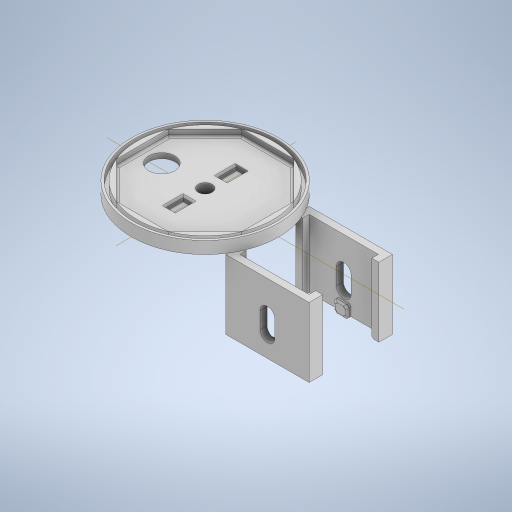
# Autodesk Inventor part: Bi_PAM
Saved by Autodesk Inventor 2024 (Build 280153000, 153)
## iProperties
Created: 2023-07-24
Part Number: Bi_PAM
Material: 일반
Document SubType Name: Modeling
Designer: jsw
Density: 1 g/cm^3
Appearance: 기본값
Author: jsw
Autodesk Inventor part; units mm, degrees
ref_plane "YZ Plane" through (0, 0, 0) normal (1, 0, 0) x (0, 1, 0)
sketch "스케치1" plane through (0, 0, 0) normal (0, 1, 0) x (-1, 0, 0)
  circle A0 centre (0, 0) radius 39
  circle A1 centre (0, 0) radius 42.5
  dimension "d0" = 78
  dimension "d6" = 3.5
  constraints: 2 centre point, 2 coincident
  measures "d0" diameter of A0
  measures "d6" radial gap between concentric circles of A0 A1
extrude "돌출1" add sketch "스케치1" along normal blind 7 contours A0 | A1
sketch "스케치4" plane through (0, 7, 0) normal (0, 1, 0) x (1, 0, 0)
  line L0 (15, -36.2132) -> (-15, -36.2132)
  line L1 (-15, -36.2132) -> (-36.2132, -15)
  line L2 (-36.2132, -15) -> (-36.2132, 15)
  line L3 (-36.2132, 15) -> (-15, 36.2132)
  line L4 (-15, 36.2132) -> (15, 36.2132)
  line L5 (15, 36.2132) -> (36.2132, 15)
  line L6 (36.2132, 15) -> (36.2132, -15)
  line L7 (36.2132, -15) -> (15, -36.2132)
  point P0 (0, 0)
  point P1 (0, 0)
  dimension "d17" = 30
  constraints: 16 end point, 1 coincident, 1 horizontal, 17 other
  measures "d17" distance of L0.start L0.end
extrude "돌출4" cut sketch "스케치4" against normal blind 4
fillet "모깎기1" radius 1.2 8 edges at (0, 3, -36.2132) (25.6066, 3, -25.6066) (36.2132, 3, 0) (25.6066, 3, 25.6066) (0, 3, 36.2132) (-25.6066, 3, 25.6066) (-36.2132, 3, 0) (-25.6066, 3, -25.6066)
sketch "스케치6" plane through (0, 7, 0) normal (0, 1, 0) x (1, 0, 0)
  line L0 (36.2132, -15) -> (36.2132, 15) projected
  circle A0 centre (0, 0) radius 39.1969
  circle A1 centre (0, 0) radius 41.1969
  dimension "d30" = 2
  constraints: 2 coincident, 1 centre point, 3 other
extrude "돌출6" cut sketch "스케치6" against normal blind 4
sketch "스케치9" plane through (0, 0, 0) normal (0, -1, 0) x (1, 0, 0)
  line L0 (80, -20) -> (40, -20)
  line L1 (40, -20) -> (40, 20)
  line L2 (40, 20) -> (80, 20)
  line L3 (80, 20) -> (80, -20)
  line L4 (80, -20) -> (40, 20) construction
  line L5 (40, -20) -> (80, 20) construction
  line L6 (84, -24) -> (36, -24)
  line L7 (36, -24) -> (36, 24)
  line L8 (36, 24) -> (84, 24)
  line L9 (84, 24) -> (84, -24)
  line L10 (84, -24) -> (36, 24) construction
  line L11 (36, -24) -> (84, 24) construction
  line L12 (0, -59.5) -> (0, 59.5) projected
  line L13 (-67.8, 0) -> (109.3, 0) projected
  point P0 (60, 0)
  point P1 (60, 0)
  dimension "d54" = 40
  dimension "d55" = 40
  dimension "d56" = 4
  dimension "d112" = 60
  dimension "d113" = 0
  constraints: 24 end point, 5 midpoint, 4 parallel, 2 horizontal, 2 perpendicular, 1 point on line
  measures "d54" distance of L1.end L2.end
  measures "d55" distance of L0.end L1.end
  measures "d56" distance between parallel lines of L2 L8
  measures "d112" distance from line of point (60, 0) L12
  measures "d113" distance from line of L13 point (60, 0)
extrude "돌출9" add sketch "스케치9" along normal blind 40 contours L3 L13 L9 L6 L7 L1 L0 | L3 L2 L1 L13 L7 L8 L9
ref_plane "작업 평면2" through (60, 0, 24) normal (1, 0, 0) x (0, 0, -1)
sketch "스케치11" plane through (36, 0, 24) normal (0, 0, 1) x (1, 0, 0)
  line L0 (24, -18.25) -> (24, -27.75) construction
  line L1 (19.75, -18.25) -> (19.75, -27.75)
  line L2 (28.25, -27.75) -> (28.25, -18.25)
  arc A0 (28.25, -18.25) -> (19.75, -18.25) centre (24, -18.25) ccw
  arc A1 (19.75, -27.75) -> (28.25, -27.75) centre (24, -27.75) ccw
  line L3 (0, 0) -> (48, 0) projected
  line L4 (48, 0) -> (0, 0) projected
  point P0 (-36, 0)
  point P1 (24, -23)
  point P2 (28.25, -23)
  point P3 (24, 0)
  point P4 (24, -32)
  point P5 (24, -14)
  dimension "d63" = 4.25
  dimension "d64" = 18
  dimension "d65" = 23
  constraints: 8 end point, 6 point on circle, 4 tangent, 3 midpoint, 2 centre point, 1 parallel, 1 vertical, 1 vertical alignment
  measures "d63" distance of point (28.25, -23) point (24, -23)
  measures "d64" distance of point (24, -32) point (24, -14)
  measures "d65" distance from line of L3 point (24, -23)
extrude "돌출11" cut sketch "스케치11" against normal up to surface (48 mm away)
sketch "스케치12" plane through (80, 0, 20) normal (0, 0, -1) x (-1, 0, 0)
  line L0 (40, -40) -> (0, -40) projected
  line L1 (16, -40) -> (24, -40)
  line L2 (24, -40) -> (24, -33)
  line L3 (24, -33) -> (16, -33)
  line L4 (16, -33) -> (16, -40)
  line L5 (15.75, -18.25) -> (15.75, -27.75) projected
  line L6 (15.75, -23) -> (24.25, -23)
  line L7 (24.25, -27.75) -> (24.25, -18.25) projected
  line L8 (40, -6) -> (0, -6)
  line L9 (24, -6) -> (24, -13)
  line L10 (24, -13) -> (16, -13)
  line L11 (16, -13) -> (16, -6)
  point P0 (80, 0)
  point P1 (20, -40)
  point P2 (20, -40)
  point P3 (24, -6)
  dimension "d68" = 8
  dimension "d69" = 7
  dimension "d70" = 0
  constraints: 18 end point, 6 symmetric about line, 4 midpoint, 2 parallel, 2 point on line, 1 horizontal, 1 perpendicular
  measures "d68" distance of L3.end L2.end
  measures "d69" distance of L1.end L2.end
  measures "d70" distance of point (20, -40) point (20, -40)
extrude "돌출12" add sketch "스케치12" along normal blind 2 contours L0 L4 L3 L2
fillet "모깎기3" radius 1 4 edges at (56, -36.5, 18) (64, -36.5, 18) (60, -33, 18) (60, -40, 18)
ref_plane "작업 평면3" through (84, 0, 0) normal (0, 0, -1) x (-1, 0, 0)
mirror "미러2" about plane through (84, 0, 0) normal (0, 0, -1) of "모깎기3", "돌출12"
sketch "스케치13" plane through (0, 3, 0) normal (0, 1, 0) x (1, 0, 0)
  line L0 (2.75, -21) -> (-2.75, -21)
  line L1 (-2.75, -21) -> (-2.75, -10)
  line L2 (-2.75, -10) -> (2.75, -10)
  line L3 (2.75, -10) -> (2.75, -21)
  line L4 (2.75, -21) -> (-2.75, -10) construction
  line L5 (-2.75, -21) -> (2.75, -10) construction
  line L6 (-35.9913, 0) -> (36.8765, 0)
  line L7 (2.75, 21) -> (-2.75, 21)
  line L8 (-2.75, 21) -> (-2.75, 10)
  line L9 (-2.75, 10) -> (2.75, 10)
  line L10 (2.75, 10) -> (2.75, 21)
  line L11 (2.75, 21) -> (-2.75, 10) construction
  line L12 (-2.75, 21) -> (2.75, 10) construction
  point P0 (0, 0)
  point P1 (0, -15.5)
  point P2 (0, -10)
  point P3 (0, 15.5)
  point P4 (0, 10)
  point P5 (0.4426, 0)
  dimension "d75" = 5.5
  dimension "d76" = 11
  dimension "d77" = 10
  dimension "d78" = 0
  constraints: 26 end point, 6 symmetric about line, 4 midpoint, 2 horizontal, 2 parallel, 1 perpendicular, 1 vertical alignment
  measures "d75" distance of L1.end L2.end
  measures "d76" distance of L0.end L1.end
  measures "d77" distance of point (0, -10) point (0, 0)
  measures "d78" vertical distance of point (0, 0) point (0.443, 0)
extrude "돌출13" cut sketch "스케치13" against normal up to surface (3 mm away)
sketch "스케치14" plane through (36, 0, -24) normal (-1, 0, 0) x (0, 0, 1)
  line L0 (66.5, 0) -> (-18.5, 0) projected
  circle A0 centre (9, -7) radius 1.25
  line L1 (24, 0) -> (24, 7)
  line L2 (9, 7) -> (39, 7) projected
  circle A1 centre (39, -7) radius 1.25
  line L3 (4, 0) -> (4, -40) projected
  line L4 (44, 0) -> (44, -40) projected
  line L5 (44, -10) -> (4, -10)
  line L6 (7.75, -10) -> (7.75, 0)
  line L7 (40.25, -10) -> (40.25, 0)
  line L8 (40.25, -10) -> (40.25, -40)
  line L9 (48, -40) -> (0, -40) projected
  line L10 (7.75, -10) -> (7.75, -40)
  point P0 (24, 0)
  dimension "d82" = 2.5
  dimension "d84" = 7
  dimension "d85" = 15
  dimension "d86" = 10
  constraints: 12 end point, 8 point on line, 3 perpendicular, 2 centre point, 2 midpoint, 2 tangent, 1 parallel, 1 symmetric about line, 1 vertical, 1 other
  measures "d82" diameter of A0
  measures "d84" distance from line of L0 A0.centre
  measures "d85" horizontal distance of L1.start A0.centre
  measures "d86" distance between parallel lines of L0 L5
extrude "돌출14" cut sketch "스케치14" against normal up to surface (48 mm away) contours A0 | A1 | L7 L5 L6 L0 | L8 L9 L10 L5
sketch "스케치15" plane through (0, 0, 0) normal (0, -1, 0) x (1, 0, 0)
  line L0 (-2.75, -21) -> (-2.75, -10) projected
  line L1 (-2.75, -10) -> (2.75, -10) projected
  line L2 (2.75, -10) -> (2.75, -21) projected
  line L3 (-2.75, 10) -> (2.75, 10) projected
  line L4 (2.75, 10) -> (2.75, 21) projected
  line L5 (-2.75, 21) -> (-2.75, 10) projected
  line L6 (2.5, 20) -> (-2.5, 20) projected
  line L7 (8.75, 21) -> (-8.75, 21)
  line L8 (-8.75, 21) -> (-8.75, -21)
  line L9 (-8.75, -21) -> (8.75, -21)
  line L10 (8.75, -21) -> (8.75, 21)
  line L11 (-2.75, 21) -> (2.75, 21) projected
  line L12 (2.75, -21) -> (-2.75, -21) projected
  point P0 (0, 0)
  point P1 (2.75, -21)
  point P2 (-2.75, 21)
  point P3 (2.75, -20.7604)
  point P4 (2.75, 21)
  point P5 (-2.75, -21)
  dimension "d89" = 6
  dimension "d90" = 6
  dimension "d115" = 0
  dimension "d116" = 0
  constraints: 6 end point, 2 horizontal, 1 parallel, 1 perpendicular, 5 other
  measures "d115" distance between parallel lines of L7 L11
  measures "d116" vertical extent of L12
extrude "돌출15" add sketch "스케치15" along normal blind 14
sketch "스케치16" plane through (8.75, 0, 19.2396) normal (1, 0, 0) x (0, 0, -1)
  circle A0 centre (4.2396, -7) radius 1.25
  line L0 (61.7396, 0) -> (-23.2604, 0) projected
  line L1 (19.2396, 0) -> (19.2396, -14)
  line L2 (40.2396, -14) -> (-1.7604, -14) projected
  circle A1 centre (34.2396, -7) radius 1.25
  point P0 (40, -14)
  point P1 (0, -14)
  dimension "d93" = 2.5
  dimension "d94" = 7
  dimension "d95" = 15
  constraints: 2 centre point, 2 end point, 2 midpoint, 1 symmetric about line, 1 other
  measures "d93" diameter of A0
  measures "d94" distance from line of L0 A0.centre
  measures "d95" horizontal distance of A0.centre L1.start
chamfer "모따기1" distance 1 angle 45 30 edges at (48, -40, -20) (72, -40, -20) (80, -40, -18.125) (80, -40, 18.125) (72, -40, 20) (48, -40, 20) (64, -40, 19.5) (63.7071, -39.7071, 18.2929) (64, -40, -19.5) (63.7071, -39.7071, -18.2929) (56.2929, -39.7071, -18.2929) (56, -40, -19.5) (56.2929, -39.7071, 18.2929) (56, -40, 19.5) (40, -40, 18.125) (40, -40, -18.125) (2.75, 3, -15.5) (0, 3, -10) (-2.75, 3, -15.5) (2.75, 3, 15.5) (-2.75, 3, 15.5) (0, 3, 10) (56.2929, -33.2929, 18.2929) (56, -33, 19.5) (63.7071, -33.2929, 18.2929) (64, -33, 19.5) (56.2929, -33.2929, -18.2929) (56, -33, -19.5) (63.7071, -33.2929, -18.2929) (64, -33, -19.5)
extrude "돌출18" cut sketch "스케치16" against normal up to surface (6 mm away)
ref_plane "작업 평면4" through (0, 0, 19.2396) normal (1, 0, 0) x (0, 0, -1)
mirror "미러3" about plane through (0, 0, 19.2396) normal (1, 0, 0) of "돌출18"
sketch "스케치18" plane through (0, -14, 0) normal (0, -1, 0) x (1, 0, 0)
  circle A0 centre (0, 0) radius 4
  dimension "d105" = 8
  constraints: 1 centre point, 1 coincident
  measures "d105" diameter of A0
extrude "돌출19" cut sketch "스케치18" against normal up to surface (17 mm away)
sketch "스케치19" plane through (0, 0, 0) normal (0, -1, 0) x (1, 0, 0)
  circle A0 centre (-25, 0) radius 7.5
  line L0 (0, -59.5) -> (0, 59.5) projected
  point P0 (0, 0)
  dimension "d108" = 15
  dimension "d114" = 25
  constraints: 1 centre point, 1 horizontal alignment
  measures "d108" diameter of A0
  measures "d114" distance from line of A0.centre L0
extrude "돌출20" cut sketch "스케치19" against normal up to surface (3 mm away)
